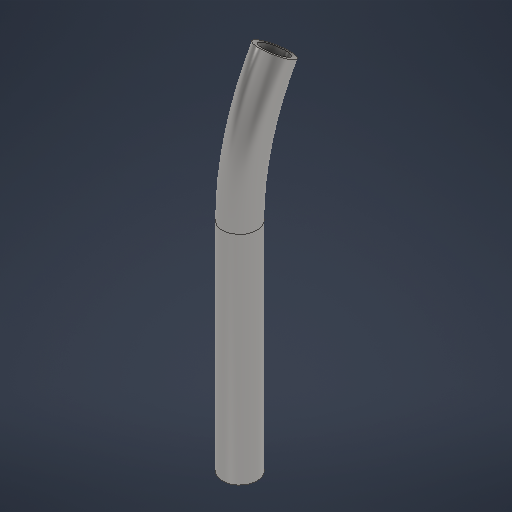
# Autodesk Inventor part: Bended shaft
Saved by Autodesk Inventor 2026.2 (Build 302298010, 298A)
## iProperties
Created: 2026-03-31
Part Number: Bended shaft
Material: Stainless Steel
Document SubType Name: Modeling
Designer: piete
Density: 8 g/cm^3
Appearance: Semi-Polished
Author: piete
Autodesk Inventor part; units mm, degrees
ref_plane "YZ Plane" through (0, 0, 0) normal (1, 0, 0) x (0, 1, 0)
ref_plane "XZ Plane" through (0, 0, 0) normal (0, 1, 0) x (-1, 0, 0)
ref_plane "XY Plane" through (0, 0, 0) normal (0, 0, 1) x (1, 0, 0)
sketch "Sketch1" plane through (0, 0, 0) normal (0, 1, 0) x (-1, 0, 0)
  circle A0 centre (0, 0) radius 4
  circle A1 centre (0, 0) radius 3
  dimension "d0" = 8
  dimension "d1" = 6
  constraints: 2 centre point, 2 coincident
  measures "d0" diameter of A0
  measures "d1" diameter of A1
extrude "Extrusion1" add sketch "Sketch1" along normal blind 50
sketch "Sketch2" plane through (0, 50, 0) normal (0, 1, 0) x (1, 0, 0)
  circle A0 centre (0, 0) radius 3
  circle A1 centre (0, 0) radius 4
  line L0 (-9.5533, 60) -> (9.0137, 60)
  dimension "d4" = 6
  dimension "d5" = 8
  dimension "d6" = 60
  constraints: 2 centre point, 2 coincident, 2 end point, 1 horizontal
  measures "d4" diameter of A0
  measures "d5" diameter of A1
  measures "d6" distance from line of L0 point (0, 0)
revolve "Revolution1" add sketch "Sketch2" angle 30 about axis through (-9.5533, 50, -60) along (-1, 0, 0)
body "Solid1"
